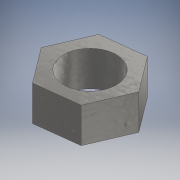
# Autodesk Inventor part: m3_nut
Saved by Autodesk Inventor 2017 (Build 210142000, 142)
## iProperties
Created: 2018-04-08
Part Number: m3_nut
Material: Steel, Galvanized
Document SubType Name: Modeling
Designer: Roland
Density: 7.85 g/cm^3
Appearance: Galvanized
Author: Roland
Autodesk Inventor part; units mm, degrees
ref_plane "YZ Plane" through (0, 0, 0) normal (1, 0, 0) x (0, 1, 0)
ref_plane "XZ Plane" through (0, 0, 0) normal (0, 1, 0) x (-1, 0, 0)
ref_plane "XY Plane" through (0, 0, 0) normal (0, 0, 1) x (1, 0, 0)
sketch "Sketch1" plane through (0, 0, 0) normal (0, 0, 1) x (1, 0, 0)
  circle A0 centre (0, 0) radius 1.5
  line L0 (-1.5, 2) -> (0.9821, 2.299)
  line L1 (0.9821, 2.299) -> (2.4821, 0.299)
  line L2 (2.4821, 0.299) -> (1.5, -2)
  line L3 (1.5, -2) -> (-0.9821, -2.299)
  line L4 (-0.9821, -2.299) -> (-2.4821, -0.299)
  line L5 (-2.4821, -0.299) -> (-1.5, 2)
  dimension "d0" = 3
  constraints: 12 end point, 2 coincident, 1 centre point, 13 other
  measures "d0" diameter of A0
extrude "Extrusion1" add sketch "Sketch1" along normal blind 2
body "Solid1"
